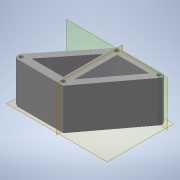
# Autodesk Inventor part: steunstuk driehoek
Saved by Autodesk Inventor 2021 (Build 250183000, 183)
## iProperties
Manager: PJ / DCS
Company: Emmaüs Bovenbouw Aalter
Created: 2021-02-03
Part Number: steunstuk driehoek
Material: S235
Catalog Web Link: http://emmausbovenbouw.op-weg.be/
Vendor: Emmaüsinstituut Bovenbouw Aalter
Document SubType Name: Modeling
Designer: Antho
Engineer: Declercq St.
Manufacturer: Standard
Standards Organization: Custom
Density: 7.86 g/cm^3
Appearance: Steel
Title: Algemene titel
Subject: Specifieke titel
Author: Antho
Keywords: Ruwe Ø xxxxx
Comments: Opmerking
Autodesk Inventor part; units mm, degrees
sketch "Sketch2" plane through (0, 0, 0) normal (0, 0, 1) x (1, 0, 0)
  line L0 (0, 2.8582) -> (0, -2.8582) construction
  line L1 (-5.7775, 0) -> (5.7775, 0) construction
  line L2 (0, 0) -> (4, 0)
  line L3 (4, 0) -> (-4, 0)
  circle A0 centre (0, 0) radius 4
  line L4 (0, 0) -> (-2, 3.4641)
  line L5 (0, 0) -> (4, 0) construction
  line L6 (0, 0) -> (2, 3.4641)
  line L7 (0, 0) -> (4, 0) construction
  line L8 (0, 0) -> (4, 0)
  line L9 (0, 0) -> (2, -3.4641)
  line L10 (0, 0) -> (-2, -3.4641)
  line L11 (-2, 3.4641) -> (2, 3.4641)
  line L12 (2, 3.4641) -> (4, 0)
  line L13 (4, 0) -> (2, -3.4641)
  line L14 (2, -3.4641) -> (-2, -3.4641)
  line L15 (-2, -3.4641) -> (-4, 0)
  line L16 (-4, 0) -> (-2, 3.4641)
  dimension "d3" = 4
  dimension "d2" = 8
  dimension "d1" = 120
  dimension "d0" = 60
  constraints: 34 end point, 5 point on circle, 4 equal length, 3 coincident, 3 horizontal, 3 point on line, 2 midpoint, 1 centre point, 1 vertical
  measures "d3" distance of L2.start L2.end
  measures "d2" distance of L2.end L3.end
  measures "d1" angle of L5 L4
  measures "d0" angle of L7 L6
extrude "Extrusion1" add sketch "Sketch2" along normal blind 43.5 contours L6 L12 L2 | L10 L15 L3 | L3 L16 L4 | L4 L11 L6 | L2 L13 L9 | L9 L14 L10
sketch "Sketch3" plane through (0, 0, 43.5) normal (0, 0, 1) x (1, 0, 0)
  point P0 (0, 0)
  point P1 (0, 0)
  constraints: 1 coincident
hole "Hole1" at (0, 0, 43.5) direction (0, 0, -1) diameter 4.2 depth 44
sketch "Sketch5" plane through (0, 0, 43.5) normal (0, 0, 1) x (1, 0, 0)
  line L0 (0, 0) -> (0, -56.314)
  line L1 (0, -56.314) -> (4, -56.314)
  line L2 (4, -56.314) -> (2, -59.7781)
  line L3 (2, -59.7781) -> (-2, -59.7781)
  line L4 (-2, -59.7781) -> (-4, -56.314)
  line L5 (0, -56.314) -> (-4, -56.314)
  line L6 (0, -56.314) -> (0, -52.85)
  line L7 (0, -52.85) -> (2, -52.85)
  line L8 (2, -52.85) -> (4, -56.314)
  line L9 (0, -52.85) -> (-2, -52.85)
  line L10 (-2, -52.85) -> (-4, -56.314)
  line L11 (4, 0) -> (4, -56.314)
  line L12 (-4, 0) -> (-2, -3.4641) projected
  line L13 (-4, 0) -> (-4, -56.314)
  line L14 (0, -56.314) -> (-44.771, -56.314)
  line L15 (-44.771, -56.314) -> (-44.771, -60.314)
  line L16 (-44.771, -56.314) -> (-44.771, -52.314)
  line L17 (-44.771, -60.314) -> (-41.307, -58.3138)
  line L18 (-44.771, -52.314) -> (-41.307, -54.3142)
  line L19 (-41.307, -54.3142) -> (-41.307, -58.3138)
  line L20 (-44.771, -60.314) -> (-48.235, -58.3138)
  line L21 (-44.771, -52.314) -> (-48.235, -54.3142)
  line L22 (-48.235, -54.3142) -> (-48.235, -58.3138)
  line L23 (-44.771, -60.314) -> (-0.654, -60.314)
  line L24 (-0.654, -60.314) -> (4, -56.314)
  line L25 (-44.771, -52.314) -> (0, -52.314)
  line L26 (-4, 0) -> (0, -3.4641)
  line L27 (-2, -3.4641) -> (2, -3.4641) projected
  line L28 (0, -3.4641) -> (4, 0)
  line L29 (4, -56.314) -> (4, -60.314)
  line L30 (4, -60.314) -> (-1.654, -60.314)
  point P0 (-4, -52.314)
  point P1 (-0.654, -60.314)
  dimension "d21" = 56.314
  dimension "d22" = 4
  dimension "d23" = 4
  dimension "d24" = 4
  dimension "d25" = 4
  dimension "d26" = 3.4641
  dimension "d27" = 3.464
  dimension "d28" = 2
  dimension "d29" = 2
  dimension "d30" = 44.771
  dimension "d31" = 4
  dimension "d35" = 4
  dimension "d38" = 4
  dimension "d39" = 3.464
  dimension "d40" = 4
  dimension "d41" = 3.464
  dimension "d42" = 4
  dimension "d43" = 4
  dimension "d44" = 3.464
  dimension "d45" = 3.464
  constraints: 58 end point, 5 horizontal, 5 point on line, 3 vertical, 2 perpendicular, 1 midpoint
  measures "d21" distance of L0.start L0.end
  measures "d22" distance of L1.end L2.end
  measures "d23" distance of L2.end L3.end
  measures "d24" distance of L4.end L3.end
  measures "d25" distance of L0.end L4.end
  measures "d26" distance between parallel lines of L5 L3
  measures "d27" distance of L0.end L6.end
  measures "d28" distance of L6.end L7.end
  measures "d29" distance of L6.end L9.end
  measures "d30" distance of L0.end L14.end
  measures "d31" distance of L14.end L15.end
  measures "d35" distance of L14.end L16.end
  measures "d38" distance of L15.end L17.end
  measures "d39" distance from line of L15 L17.end
  measures "d40" distance of L16.end L18.end
  measures "d41" distance from line of L16 L18.end
  measures "d42" distance of L15.end L20.end
  measures "d43" distance of L16.end L21.end
  measures "d44" distance from line of L16 L21.end
  measures "d45" distance from line of L15 L20.end
extrude "Extrusion2" add sketch "Sketch5" against normal blind 43.5
sketch "Sketch6" plane through (0, 0, 43.5) normal (0, 0, 1) x (1, 0, 0)
  circle A0 centre (0, 0) radius 1.7294 projected
  line L0 (0, 0) -> (0, -56.314)
  line L1 (0, -56.314) -> (-44.771, -56.314)
  line L2 (-4, -52.314) -> (-44.771, -52.314) projected
  dimension "d74" = 44.771
  dimension "d75" = 4
  constraints: 4 end point, 2 coincident, 1 horizontal, 1 vertical
  measures "d74" distance of L1.start L1.end
  measures "d75" distance between parallel lines of L2 L1
hole "Hole3" at (0, -56.314, 43.5) at (-44.771, -56.314, 43.5) direction (0, 0, -1) diameter 4.2 depth 44
sketch "Sketch8" plane through (0, 0, 43.5) normal (0, 0, 1) x (1, 0, 0)
  circle A0 centre (0, 0) radius 2.1 projected
  line L0 (0, 0) -> (44.771, 0)
  line L1 (44.771, 0) -> (48.771, 0)
  line L2 (44.771, 0) -> (44.771, 3.464)
  line L3 (44.771, 3.464) -> (46.771, 3.464)
  line L4 (46.771, 3.464) -> (48.771, 0)
  line L5 (44.771, 0) -> (44.771, -3.464)
  line L6 (44.771, -3.464) -> (46.771, -3.464)
  line L7 (46.771, -3.464) -> (48.771, 0)
  line L8 (44.771, 0) -> (40.771, 0)
  line L9 (44.771, -3.464) -> (42.771, -3.464)
  line L10 (42.771, -3.464) -> (40.771, 0)
  line L11 (44.771, 3.464) -> (42.771, 3.464)
  line L12 (42.771, 3.464) -> (40.771, 0)
  line L13 (2, 3.4641) -> (-2, 3.4641) projected
  line L14 (2, 3.4641) -> (44.771, 3.464)
  line L15 (44.771, -3.464) -> (4, -3.464)
  line L16 (4, -60.314) -> (4, 0) projected
  line L17 (4, -3.464) -> (2, 3.4641)
  dimension "d62" = 44.771
  dimension "d63" = 4
  dimension "d64" = 3.464
  dimension "d65" = 2
  dimension "d66" = 3.464
  dimension "d67" = 2
  dimension "d68" = 4
  dimension "d69" = 2
  dimension "d70" = 2
  constraints: 32 end point, 4 point on line, 3 horizontal, 2 perpendicular, 1 parallel, 1 vertical
  measures "d62" distance of L0.start L0.end
  measures "d63" distance of L0.end L1.end
  measures "d64" distance of L0.end L2.end
  measures "d65" distance of L2.end L3.end
  measures "d66" distance of L0.end L5.end
  measures "d67" distance of L5.end L6.end
  measures "d68" distance of L0.end L8.end
  measures "d69" distance of L5.end L9.end
  measures "d70" distance of L2.end L11.end
extrude "Extrusion3" add sketch "Sketch8" against normal blind 43.5 contours L17 L14 L12 L0 | L0 L16 L17 | L0 L10 L15 L16 | L12 L11 L2 L0 | L0 L5 L9 L10 | L2 L3 L4 L1 | L1 L7 L6 L5
sketch "Sketch9" plane through (0, 0, 43.5) normal (0, 0, 1) x (1, 0, 0)
  line L0 (0, 0) -> (44.771, 0)
  dimension "d73" = 44.771
  constraints: 2 end point, 1 coincident, 1 horizontal
  measures "d73" distance of L0.start L0.end
hole "Hole5" at (44.771, 0, 43.5) direction (0, 0, -1) diameter 4.2 depth 44
sketch "Sketch10" plane through (0, 0, 43.5) normal (0, 0, 1) x (1, 0, 0)
  line L0 (4, -3.464) -> (4, -60.314) projected
  line L1 (46.771, -3.464) -> (4, -3.464) projected
  line L2 (4, -60.314) -> (46.771, -3.464)
  line L3 (21.4983, -3.464) -> (21.4983, 3.4641)
  line L4 (2, 3.4641) -> (46.771, 3.464) projected
  line L5 (43.6374, -7.6291) -> (38.1012, -3.464)
  line L6 (38.1012, -3.464) -> (4, -48.7904)
  line L7 (38.1012, -3.464) -> (38.1012, -3.464)
  line L8 (38.1012, -3.464) -> (46.771, -3.464)
  line L9 (4, -48.7904) -> (4, -60.314)
  line L10 (-2, 3.4641) -> (-4, 0) projected
  line L11 (-48.235, -54.3142) -> (-44.771, -52.314) projected
  line L12 (-2, 3.4641) -> (-48.235, -54.3142)
  line L13 (-33.3199, -35.6753) -> (-27.9106, -40.0039)
  line L14 (-27.9106, -40.0039) -> (-4, -10.1236)
  line L15 (-4, -52.314) -> (-4, 0) projected
  line L16 (2, 3.4641) -> (-2, 3.4641) projected
  line L17 (-4, -10.1236) -> (-2, 3.4641)
  line L18 (-27.9106, -40.0039) -> (-37.7613, -52.314)
  line L19 (-37.7613, -52.314) -> (-48.235, -54.3142)
  point P0 (0, 0)
  dimension "d83" = 6.9281
  dimension "d84" = 6.928
  dimension "d85" = 6.928
  dimension "d86" = 90
  dimension "d87" = 90
  dimension "d88" = 90
  dimension "d89" = 90
  dimension "d90" = 90
  constraints: 26 end point, 8 point on line, 2 perpendicular, 1 collinear, 1 horizontal, 1 vertical
  measures "d83" distance of L3.start L3.end
  measures "d84" distance of L5.start L5.end
  measures "d85" distance of L13.start L13.end
  measures "d86" angle of L12 L13
  measures "d87" angle of L13 L14
  measures "d88" angle of L13 L18
  measures "d89" angle of L5 L2
  measures "d90" angle of L7 L5
extrude "Extrusion4" add sketch "Sketch10" against normal blind 43.5 contours L17 L15 L10 | L10 L15 L14 L13 L12 | L6 L5 L2 L0 | L1 L2 L5 | L13 L18 L19 L12
body "Solid1"
